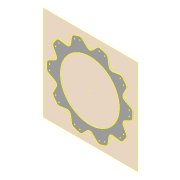
# Autodesk Inventor part: Anglerfish_3inch_tube_rubberring
Saved by Autodesk Inventor 2022 (Build 260153000, 153)
## iProperties
Created: 2022-04-17
Part Number: Anglerfish_3inch_tube_rubberring
Material: Generic
Document SubType Name: Modeling
Designer: Prakash Lab
Density: 1 g/cm^3
Appearance: Default
Author: Prakash Lab
Autodesk Inventor part; units mm, degrees
ref_plane "YZ Plane" through (0, 0, 0) normal (1, 0, 0) x (0, 1, 0)
ref_plane "XZ Plane" through (0, 0, 0) normal (0, 1, 0) x (-1, 0, 0)
ref_plane "XY Plane" through (0, 0, 0) normal (0, 0, 1) x (1, 0, 0)
ref_plane "Work Plane1" through (0, 0, -4) normal (0, 0, 1) x (1, 0, 0)
sketch "Sketch1" plane through (0, 0, -4) normal (0, 0, 1) x (1, 0, 0)
  circle A0 centre (0.1176, -0.1618) radius 38.1 projected
  circle A1 centre (0, 0) radius 43.6 projected
  circle A2 centre (0, 0) radius 55.6 projected
  point P0 (0, 0)
extrude "Extrusion1" add sketch "Sketch1" along normal blind 1 contours A1 | A2
sketch "Sketch2" plane through (0, 0, -3) normal (0, 0, 1) x (1, 0, 0)
  circle A0 centre (47.1724, 15.3272) radius 2 projected
  circle A1 centre (47.1724, 15.3272) radius 4.4912
  line L0 (45.1335, 11.3256) -> (55.2569, 6.1675)
  circle A2 centre (0, 0) radius 55.6 projected
  line L1 (43.1708, 17.3662) -> (48.3289, 27.4896)
  line L2 (47.1724, 15.3272) -> (52.8787, 17.1813)
  point P0 (0, 0)
  dimension "d2" = 45
  dimension "d3" = 45
  constraints: 6 end point, 5 point on circle, 2 tangent, 1 centre point, 1 line through centre
  measures "d2" angle of L2 L1
  measures "d3" angle of L2 L0
extrude "Extrusion2" cut sketch "Sketch2" against normal blind 1 contours A0 | A1 | A1 L1 A2 L2 | L2 A2 L0 A1
fillet "Fillet1" radius 4 2 edges at (48.3289, 27.4896, -3.5) (55.2569, 6.1675, -3.5)
pattern_circular "Circular Pattern1" count 10 over 360 about axis through (0, 0, -4) along (0, 0, 1) of "Extrusion2", "Fillet1"
sketch "Sketch3" plane through (0, 0, -3) normal (0, 0, 1) x (1, 0, 0)
  arc A0 (47.1551, -29.4578) -> (47.3266, -25.5226) centre (43.7626, -27.3385) ccw projected
  line L0 (47.3266, -25.5226) -> (43.1708, -17.3662) projected
  arc A1 (45.1335, -11.3256) -> (43.1708, -17.3662) centre (47.1724, -15.3272) ccw projected
  line L1 (45.1335, -11.3256) -> (53.2898, -7.1697) projected
  arc A2 (53.2898, -7.1697) -> (55.4641, -3.8852) centre (51.4739, -3.6057) ccw projected
  arc A3 (55.4641, -3.8852) -> (55.4641, 3.8852) centre (0, 0) ccw projected
  arc A4 (55.4641, 3.8852) -> (53.2898, 7.1697) centre (51.4739, 3.6057) ccw projected
  line L2 (53.2898, 7.1697) -> (45.1335, 11.3256) projected
  arc A5 (43.1708, 17.3662) -> (45.1335, 11.3256) centre (47.1724, 15.3272) ccw projected
  line L3 (43.1708, 17.3662) -> (47.3266, 25.5226) projected
  arc A6 (47.3266, 25.5226) -> (47.1551, 29.4578) centre (43.7626, 27.3385) ccw projected
  arc A7 (47.1551, 29.4578) -> (42.5877, 35.7442) centre (0, 0) ccw projected
  arc A8 (42.5877, 35.7442) -> (38.8981, 37.1234) centre (39.5239, 33.1726) ccw projected
  line L4 (38.8981, 37.1234) -> (29.8567, 35.6914) projected
  arc A9 (24.7183, 39.4247) -> (29.8567, 35.6914) centre (29.1541, 40.1272) ccw projected
  line L5 (24.7183, 39.4247) -> (23.2863, 48.4661) projected
  arc A10 (23.2863, 48.4661) -> (20.8344, 51.5489) centre (19.3355, 47.8403) ccw projected
  arc A11 (20.8344, 51.5489) -> (13.4443, 53.9501) centre (0, 0) ccw projected
  arc A12 (13.4443, 53.9501) -> (9.6487, 52.8972) centre (12.4771, 50.0688) ccw projected
  line L6 (9.6487, 52.8972) -> (3.1757, 46.4243) projected
  arc A13 (-3.1757, 46.4243) -> (3.1757, 46.4243) centre (0, 49.6) ccw projected
  line L7 (-3.1757, 46.4243) -> (-9.6487, 52.8972) projected
  arc A14 (-9.6487, 52.8972) -> (-13.4443, 53.9501) centre (-12.4771, 50.0688) ccw projected
  arc A15 (-13.4443, 53.9501) -> (-20.8344, 51.5489) centre (0, 0) ccw projected
  arc A16 (-20.8344, 51.5489) -> (-23.2863, 48.4661) centre (-19.3355, 47.8403) ccw projected
  line L8 (-23.2863, 48.4661) -> (-24.7183, 39.4247) projected
  arc A17 (-29.8567, 35.6914) -> (-24.7183, 39.4247) centre (-29.1541, 40.1272) ccw projected
  line L9 (-29.8567, 35.6914) -> (-38.8981, 37.1234) projected
  arc A18 (-38.8981, 37.1234) -> (-42.5877, 35.7442) centre (-39.5239, 33.1726) ccw projected
  arc A19 (-42.5877, 35.7442) -> (-47.1551, 29.4578) centre (0, 0) ccw projected
  arc A20 (-47.1551, 29.4578) -> (-47.3266, 25.5226) centre (-43.7626, 27.3385) ccw projected
  line L10 (-47.3266, 25.5226) -> (-43.1708, 17.3662) projected
  arc A21 (-45.1335, 11.3256) -> (-43.1708, 17.3662) centre (-47.1724, 15.3272) ccw projected
  line L11 (-45.1335, 11.3256) -> (-53.2898, 7.1697) projected
  arc A22 (-53.2898, 7.1697) -> (-55.4641, 3.8852) centre (-51.4739, 3.6057) ccw projected
  arc A23 (-55.4641, 3.8852) -> (-55.4641, -3.8852) centre (0, 0) ccw projected
  arc A24 (-55.4641, -3.8852) -> (-53.2898, -7.1697) centre (-51.4739, -3.6057) ccw projected
  line L12 (-53.2898, -7.1697) -> (-45.1335, -11.3256) projected
  arc A25 (-43.1708, -17.3662) -> (-45.1335, -11.3256) centre (-47.1724, -15.3272) ccw projected
  line L13 (-43.1708, -17.3662) -> (-47.3266, -25.5226) projected
  arc A26 (-47.3266, -25.5226) -> (-47.1551, -29.4578) centre (-43.7626, -27.3385) ccw projected
  arc A27 (-47.1551, -29.4578) -> (-42.5877, -35.7442) centre (0, 0) ccw projected
  arc A28 (-42.5877, -35.7442) -> (-38.8981, -37.1234) centre (-39.5239, -33.1726) ccw projected
  line L14 (-38.8981, -37.1234) -> (-29.8567, -35.6914) projected
  arc A29 (-24.7183, -39.4247) -> (-29.8567, -35.6914) centre (-29.1541, -40.1272) ccw projected
  line L15 (-24.7183, -39.4247) -> (-23.2863, -48.4661) projected
  arc A30 (-23.2863, -48.4661) -> (-20.8344, -51.5489) centre (-19.3355, -47.8403) ccw projected
  arc A31 (-20.8344, -51.5489) -> (-13.4443, -53.9501) centre (0, 0) ccw projected
  arc A32 (-13.4443, -53.9501) -> (-9.6487, -52.8972) centre (-12.4771, -50.0688) ccw projected
  line L16 (-9.6487, -52.8972) -> (-3.1757, -46.4243) projected
  arc A33 (3.1757, -46.4243) -> (-3.1757, -46.4243) centre (0, -49.6) ccw projected
  line L17 (3.1757, -46.4243) -> (9.6487, -52.8972) projected
  arc A34 (9.6487, -52.8972) -> (13.4443, -53.9501) centre (12.4771, -50.0688) ccw projected
  arc A35 (13.4443, -53.9501) -> (20.8344, -51.5489) centre (0, 0) ccw projected
  arc A36 (20.8344, -51.5489) -> (23.2863, -48.4661) centre (19.3355, -47.8403) ccw projected
  line L18 (23.2863, -48.4661) -> (24.7183, -39.4247) projected
  arc A37 (29.8567, -35.6914) -> (24.7183, -39.4247) centre (29.1541, -40.1272) ccw projected
  line L19 (29.8567, -35.6914) -> (38.8981, -37.1234) projected
  arc A38 (38.8981, -37.1234) -> (42.5877, -35.7442) centre (39.5239, -33.1726) ccw projected
  arc A39 (42.5877, -35.7442) -> (47.1551, -29.4578) centre (0, 0) ccw projected
  circle A40 centre (0.1176, -0.1618) radius 38.1 projected
  point P0 (0, 0)
equation "\"d3\" = d2"
body "Solid1"
